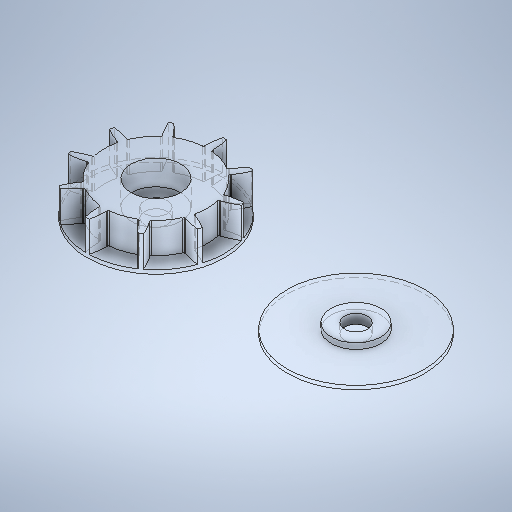
# Autodesk Inventor part: bearingear10
Saved by Autodesk Inventor 2025.2 (Build 292293000, 293)
## iProperties
Created: 2025-02-13
Part Number: bearingear10
Material: Generic
Document SubType Name: Modeling
Designer: Teamaerosal
Density: 1 g/cm^3
Appearance: Default
Author: Teamaerosal
Autodesk Inventor part; units mm, degrees
ref_plane "YZ Plane" through (0, 0, 0) normal (1, 0, 0) x (0, 1, 0)
ref_plane "XZ Plane" through (0, 0, 0) normal (0, 1, 0) x (-1, 0, 0)
ref_plane "XY Plane" through (0, 0, 0) normal (0, 0, 1) x (1, 0, 0)
sketch "Sketch1" plane through (0, 0, 0) normal (0, 1, 0) x (-1, 0, 0)
  circle A0 centre (0, 0) radius 18
  circle A1 centre (0, 0) radius 16.7855
  circle A2 centre (0, 0) radius 13.999
  line L0 (0, -13.999) -> (0, 0) construction
  line L1 (0, 0) -> (13.999, 0) construction
  circle A3 centre (0, 0) radius 13.5
  arc A4 (0.5001, -17.9931) -> (1, -13.9632) centre (-19.096, -13.5161) ccw
  arc A5 (-1, -13.9632) -> (-0.5001, -17.9931) centre (19.096, -13.5161) ccw
  line L2 (-1, -13.9632) -> (-1, -13.4629)
  line L3 (1, -13.9632) -> (1, -13.4629)
  circle A6 centre (0, 0) radius 3
  circle A7 centre (0, 0) radius 6.5
  circle A8 centre (-52.3581, 0.013) radius 18
  circle A9 centre (-52.3581, 0.013) radius 16.7855
  circle A10 centre (-52.3581, 0.013) radius 13.999
  line L4 (-52.3581, -13.986) -> (-52.3581, 0.013) construction
  line L5 (-52.3581, 0.013) -> (-38.3591, 0.013) construction
  circle A11 centre (-52.3581, 0.013) radius 13.5
  arc A12 (-51.858, -17.98) -> (-51.3581, -13.9502) centre (-71.4541, -13.5031) ccw
  arc A13 (-53.3581, -13.9502) -> (-52.8582, -17.98) centre (-33.2621, -13.5031) ccw
  line L6 (-53.3581, -13.9502) -> (-53.3581, -13.4499)
  line L7 (-51.3581, -13.9502) -> (-51.3581, -13.4499)
  circle A14 centre (-52.3581, 0.013) radius 3
  circle A15 centre (-52.3581, 0.013) radius 6.5
  point P0 (0, -16.7855)
  point P1 (0, -16.7855)
  point P2 (0.74, -16.7692)
  point P3 (-0.74, -16.7692)
  point P4 (-0.4999, -17.9931)
  point P5 (-3.765, -17.6018)
  point P6 (0.5138, -17.9927)
  point P7 (-0.5138, -17.9927)
  point P8 (0, -18)
  point P9 (-1, -13.9632)
  point P10 (-0.5001, -17.9931)
  point P11 (1.25, 0)
  point P12 (-52.3581, -16.7725)
  point P13 (-52.3581, -16.7725)
  point P14 (-51.6181, -16.7561)
  point P15 (-53.0981, -16.7561)
  point P16 (-52.858, -17.98)
  point P17 (-56.1231, -17.5888)
  point P18 (-51.8443, -17.9796)
  point P19 (-52.8719, -17.9796)
  point P20 (-52.3581, -17.987)
  point P21 (-53.3581, -13.9502)
  point P22 (-51.1081, 0.013)
  dimension "d0" = 36
  dimension "d1" = 33.571
  dimension "d2" = 27.998
  dimension "d3" = 1.48
  dimension "d4" = 27
  dimension "d13" = 20.101
  dimension "d14" = 1
  dimension "d16" = 1
  dimension "d17" = 4.001
  dimension "d18" = 1.2239
  dimension "d19" = 2.7702
  dimension "d23" = 0.5003
  dimension "d24" = 0.5003
  dimension "d42" = 6
  dimension "d43" = 13
  dimension "d48" = 36
  dimension "d49" = 33.571
  dimension "d50" = 27.998
  dimension "d51" = 1.48
  dimension "d52" = 27
  dimension "d53" = 20.101
  dimension "d54" = 1
  dimension "d55" = 1
  dimension "d56" = 4.001
  dimension "d57" = 1.2239
  dimension "d58" = 2.7702
  dimension "d59" = 0.5003
  dimension "d60" = 0.5003
  dimension "d61" = 6
  dimension "d62" = 13
  constraints: 42 point on circle, 16 centre point, 16 coincident, 16 end point, 6 symmetric about line, 6 vertical, 2 horizontal alignment, 2 perpendicular, 2 vertical alignment, 2 other
  measures "d0" diameter of A0
  measures "d1" diameter of A1
  measures "d2" diameter of A2
  measures "d3" distance of point (0.74, -16.769) point (-0.74, -16.769)
  measures "d4" diameter of A3
  measures "d13" radius of A4
  measures "d14" distance from line of L3.start L0
  measures "d16" distance of A0.end A0.start
  measures "d17" distance of point (0, -18) point (0, -13.999)
  measures "d18" vertical distance of point (-0.74, -16.769) A0.start
  measures "d19" vertical distance of point (-0.74, -16.769) L0.start
  measures "d23" distance of L3.end L3.start
  measures "d24" distance of L2.end point (-1, -13.963)
  measures "d42" diameter of A6
  measures "d43" diameter of A7
  measures "d48" diameter of A8
  measures "d49" diameter of A9
  measures "d50" diameter of A10
  measures "d51" distance of point (-51.618, -16.756) point (-53.098, -16.756)
  measures "d52" diameter of A11
  measures "d53" radius of A12
  measures "d54" distance from line of L7.start L4
  measures "d55" distance of A12.start A8.start
  measures "d56" distance of point (-52.358, -17.987) point (-52.358, -13.986)
  measures "d57" vertical distance of point (-53.098, -16.756) A8.start
  measures "d58" vertical distance of point (-53.098, -16.756) L4.start
  measures "d59" distance of L7.end L7.start
  measures "d60" distance of L6.end point (-53.358, -13.95)
  measures "d61" diameter of A14
  measures "d62" diameter of A15
extrude "Extrusion1" add sketch "Sketch1" along normal blind 8 contours A5 A1 A4 A0 | A5 A2 A4 A1 | L2 A3 L3 A2 | A3 | A6 | A7 picked at (-0.0822, -17.3191) picked at (-0.2901, -15.2142) picked at (0.7779, -13.6407)
fillet "Fillet1" radius 0.3 2 edges at (1, 4, -13.4629) (-1, 4, -13.4629)
pattern_circular "Circular Pattern1" count 10 over 360 about axis through (0, 0, 0) along (0, 1, 0) of "Extrusion1", "Fillet1"
extrude "Extrusion2" cut sketch "Sketch1" along normal blind 8 contours A6
extrude "Extrusion5" cut sketch "Sketch1" along normal blind 8 contours A7
extrude "Extrusion3" add sketch "Sketch1" against normal blind 1 contours A0 A4 A1 A5 | A5 A1 A4 A0 | A5 A2 A4 A1 | A1 A4 A2 A5 | L2 A3 L3 A2 | A2 L3 A3 L2 | A3 | A7 | A8 A12 A9 A13 | A13 A9 A12 A8 | A13 A10 A12 A9 | A9 A12 A10 A13 | L6 A11 L7 A10 | A10 L7 A11 L6 | A11 | A15
extrude "Extrusion6" add sketch "Sketch1" along normal blind 1.5 contours A7 | A15
sketch "Sketch2" plane through (52.3581, 0, 0.013) normal (0, 1, 0) x (1, 0, 0)
  point P0 (-52.3581, 0.013)
body "Solid1"
